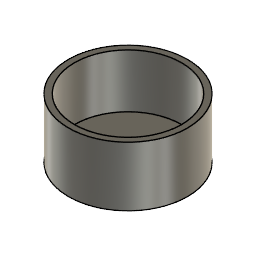
Box (Autodesk Fusion 360 design; units mm, degrees)
Autodesk Fusion 360 part; units mm, degrees
cylinder "Grundkörper Zylinder1" add diameter 50 height 25 placed x (1, 0, 0) y (0, 1, 0) z (0, 0, 1) at (0, 0, 0)
shell "Schale1" thickness 2.5 removed faces 1 at (-6.7759, -1.242, 25)
